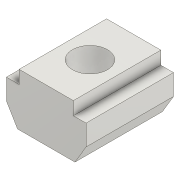
# Autodesk Inventor part: 20x20_nut
Saved by Autodesk Inventor 2020.1 (Build 241239000, 239)
## iProperties
Created: 2020-02-17
Part Number: 20x20_nut
Material: Steel, Wrought
Document SubType Name: Modeling
Designer: kuzmin
Density: 7.85 g/cm^3
Appearance: Steel
Author: kuzmin
Autodesk Inventor part; units mm, degrees
ref_plane "YZ Plane" through (0, 0, 0) normal (1, 0, 0) x (0, 1, 0)
ref_plane "XZ Plane" through (0, 0, 0) normal (0, 1, 0) x (-1, 0, 0)
ref_plane "XY Plane" through (0, 0, 0) normal (0, 0, 1) x (1, 0, 0)
sketch "Sketch1" plane through (0, 0, 0) normal (0, 0, 1) x (1, 0, 0)
  line L0 (-3.2808, -3.1442) -> (3.2808, -3.1442)
  line L1 (3.2808, -3.1442) -> (4.55, -1.0096)
  line L2 (4.55, -1.0096) -> (4.55, 1.3558)
  line L3 (4.55, 1.3558) -> (3.1, 1.3558)
  line L4 (3.1, 1.3558) -> (3.1, 2.8558)
  line L5 (3.1, 2.8558) -> (-3.1, 2.8558)
  line L6 (-3.1, 2.8558) -> (-3.1, 1.3558)
  line L7 (-3.1, 1.3558) -> (-4.55, 1.3558)
  line L8 (-4.55, 1.3558) -> (-4.55, -1.0096)
  line L9 (-4.55, -1.0096) -> (-3.2808, -3.1442)
  line L10 (0, -4.906) -> (0, 6.6764) construction
  line L11 (-3.1, 1.3558) -> (3.1, 1.3558) construction
  point P0 (0, 0)
  point P1 (0, 2.8558)
  point P2 (0, -3.1442)
  dimension "d0" = 6
  dimension "d1" = 4.5
  dimension "d2" = 6.2
  dimension "d3" = 9.1
  constraints: 24 end point, 6 perpendicular, 5 point on line, 2 equal length, 2 horizontal, 2 midpoint, 1 vertical
  measures "d0" distance between parallel lines of L0 L5
  measures "d1" distance between parallel lines of L0 L3
  measures "d2" distance of L4.end L5.end
  measures "d3" distance between parallel lines of L2 L8
extrude "Extrusion1" add sketch "Sketch1" along normal mid plane 10
sketch "Sketch2" plane through (-3.1, 2.8558, 5) normal (0, 1, 0) x (1, 0, 0)
  circle A0 centre (3.1, 5) radius 2
  dimension "d6" = 4
  constraints: 1 centre point, 1 coincident
  measures "d6" diameter of A0
extrude "Extrusion2" cut sketch "Sketch2" against normal blind 5
body "Solid1"
